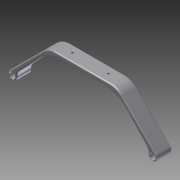
# Autodesk Inventor part: LandingBracket
Saved by Autodesk Inventor 2011 SP1 (Build 150282100, 282)
## iProperties
Created: 2011-08-02
Part Number: LandingBracket
Document SubType Name: Modeling
Designer: Nathan
Density: 1 g/cm^3
Author: Nathan
Autodesk Inventor part; units mm, degrees
ref_plane "YZ Plane" through (0, 0, 0) normal (1, 0, 0) x (0, 1, 0)
ref_plane "XZ Plane" through (0, 0, 0) normal (0, 1, 0) x (-1, 0, 0)
ref_plane "XY Plane" through (0, 0, 0) normal (0, 0, 1) x (1, 0, 0)
sketch "Sketch1" plane through (0, 0, 0) normal (0, 0, 1) x (1, 0, 0)
  line L0 (0, -9.9143) -> (0, 12.2343)
  line L1 (-107.95, 0) -> (-50.8, 57.15)
  line L2 (-50.8, 57.15) -> (0, 57.15)
  line L3 (0, 50.8) -> (-50.8, 50.8)
  line L4 (-50.8, 50.8) -> (-98.9319, 0)
  line L5 (-26.3399, 0) -> (16.21, 0)
  arc A0 (-107.95, 0) -> (-98.9319, 0) centre (-103.4409, -4.5091) ccw
  line L6 (107.95, 0) -> (50.8, 57.15)
  line L7 (50.8, 57.15) -> (0, 57.15)
  line L8 (0, 50.8) -> (50.8, 50.8)
  line L9 (50.8, 50.8) -> (98.9319, 0)
  arc A1 (98.9319, 0) -> (107.95, 0) centre (103.4409, -4.5091) ccw
  circle A2 centre (-103.4409, -4.5091) radius 4.7625
  circle A3 centre (103.4409, -4.5091) radius 4.7625
  point P0 (0, 0)
  dimension "d0" = 6.35
  dimension "d1" = 50.8
  dimension "d2" = 50.8
  dimension "d3" = 50.8
  dimension "d5" = 57.15
  dimension "d8" = 135
  dimension "d16" = 9.525
  dimension "d17" = 9.525
  constraints: 20 end point, 5 symmetric about line, 4 centre point, 4 point on circle, 2 coincident, 2 point on line, 2 vertical, 1 parallel, 1 perpendicular, 1 tangent, 2 other
  measures "d0" distance between parallel lines of L2 L3
  measures "d1" distance between parallel lines of L5 L3
  measures "d2" distance of L3.start L3.end
  measures "d3" distance of L1.end L2.end
  measures "d5" horizontal distance of L1.start L1.end
  measures "d8" angle of L2 L1
  measures "d16" diameter of A2
  measures "d17" diameter of A3
extrude "Extrusion2" add sketch "Sketch1" along normal blind 22.86
fillet "Fillet5" radius 44.45 1 edges at (-50.8, 50.8, 11.43)
fillet "Fillet6" radius 44.45 1 edges at (50.8, 50.8, 11.43)
fillet "Fillet7" radius 25.4 1 edges at (-50.8, 57.15, 11.43)
fillet "Fillet8" radius 25.4 1 edges at (50.8, 57.15, 11.43)
fillet "Fillet9" radius 14.2875 1 edges at (-98.9319, 0, 11.43)
fillet "Fillet10" radius 14.2875 1 edges at (98.9319, 0, 11.43)
fillet "Fillet11" radius 1.905 16 edges at (-83.0947, 24.8553, 0) (-49.9991, 55.2165, 0) (20.1395, 57.15, 0) (-20.1395, 57.15, 0) (49.9991, 55.2165, 0) (83.0947, 24.8553, 0) (105.7708, -10.445, 0) (96.1599, 1.3028, 0) (78.5558, 21.5056, 0) (49.2445, 47.1834, 0) (15.8411, 50.8, 0) (-15.8411, 50.8, 0) (-49.2445, 47.1834, 0) (-78.5558, 21.5056, 0) (-96.1599, 1.3028, 0) (-105.7708, -10.445, 0)
fillet "Fillet12" radius 1.905 14 edges at (-83.0947, 24.8553, 22.86) (-49.9991, 55.2165, 22.86) (0, 57.15, 22.86) (49.9991, 55.2165, 22.86) (83.0947, 24.8553, 22.86) (105.7708, -10.445, 22.86) (96.1599, 1.3028, 22.86) (78.5558, 21.5056, 22.86) (49.2445, 47.1834, 22.86) (0, 50.8, 22.86) (-49.2445, 47.1834, 22.86) (-78.5558, 21.5056, 22.86) (-96.1599, 1.3028, 22.86) (-105.7708, -10.445, 22.86)
sketch "Sketch2" plane through (-40.279, 57.15, 1.905) normal (0, 1, 0) x (1, 0, 0)
  line L0 (80.558, -19.05) -> (0, -19.05) projected
  line L1 (0, 0) -> (80.558, 0) projected
  line L2 (40.279, 0) -> (40.279, -19.05)
  point P0 (40.279, 1.905)
  point P1 (66.8696, -9.0369)
  point P2 (13.6884, -9.0369)
  dimension "d28" = 53.1812
  constraints: 2 end point, 2 midpoint, 1 symmetric about line
  measures "d28" distance of point (13.688, -9.037) point (66.87, -9.037)
hole "Hole1" at (26.5906, 57.15, 10.9419) at (-26.5906, 57.15, 10.9419) direction (0, -1, 0) diameter 2.6416 depth 25.4 tip angle 118 thread size "6-32 UNC" class "2B" standard "ANSI Unified Screw Threads"
body "Solid2"
